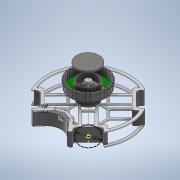
# Autodesk Inventor part: main_robot_backup
Saved by Autodesk Inventor 2020 (Build 240168000, 168)
## iProperties
Created: 2023-10-28
Part Number: main_robot_backup
Material: Типовые
Document SubType Name: Modeling
Designer: denis
Density: 1 g/cm^3
Appearance: По умолчанию
Mass: 193.225 g
Surface Area: 1128.99 cm^2
Volume: 193.225 cm^3
Author: denis
Autodesk Inventor part; units mm, degrees
(part 1 of 3)
sketch "bottom_frame" plane through (0, 0, 0) normal (0, 1, 0) x (-1, 0, 0)
  arc A0 (48.7014, 93.0224) -> (45.42, 94.668) centre (0, 0) ccw
  line L0 (0, 0) -> (74.2462, 74.2462) construction
  line L1 (85.2064, 46.3155) -> (87.5645, 48.6736)
  arc A1 (73.8927, 46.3155) -> (85.2064, 46.3155) centre (79.5495, 51.9723) ccw
  circle A2 centre (0, 0) radius 35 construction
  arc A3 (85.2064, -46.3155) -> (73.8927, -46.3155) centre (79.5495, -51.9723) ccw
  line L2 (85.2064, -46.3155) -> (87.5645, -48.6736)
  arc A4 (92.5543, -49.5852) -> (92.5543, 49.5852) centre (0, 0) ccw
  arc A5 (-46.3155, 73.8927) -> (-46.3155, 85.2064) centre (-51.9723, 79.5495) ccw
  line L3 (-48.6736, 87.5645) -> (-46.3155, 85.2064)
  arc A6 (-45.42, 94.668) -> (-48.7014, 93.0224) centre (0, 0) ccw
  arc A7 (46.3155, 85.2064) -> (46.3155, 73.8927) centre (51.9723, 79.5495) ccw
  line L4 (48.6736, 87.5645) -> (46.3155, 85.2064)
  arc A8 (44.0271, 95.3237) -> (43.577, 95.5303) centre (0, 0) ccw construction
  line L5 (46.3155, 73.8927) -> (73.8927, 46.3155)
  spline S0 degree 2 poles (87.5645, 48.6736) (91.1, 52.2091) (92.5543, 49.5852) knots 1 1 1 2 2 2
  line L6 (87.5645, 48.6736) -> (91.1, 52.2091) construction
  line L7 (91.1, 52.2091) -> (92.5543, 49.5852) construction
  line L8 (91.1, 52.2091) -> (87.5645, 48.6736) construction
  line L9 (87.5645, 48.6736) -> (91.1, 52.2091) construction
  line L10 (91.1, 52.2091) -> (92.5543, 49.5852) construction
  line L11 (91.1, 52.2091) -> (52.2091, 91.1) construction
  line L12 (52.2091, 91.1) -> (48.6736, 87.5645) construction
  line L13 (52.2091, 91.1) -> (48.6736, 87.5645) construction
  line L14 (48.6736, 87.5645) -> (52.2091, 91.1) construction
  spline S1 degree 2 poles (48.6736, 87.5645) (52.2091, 91.1) (48.7014, 93.0224) knots 1 1 1 2 2 2
  line L15 (52.2091, 91.1) -> (48.7014, 93.0224) construction
  line L16 (52.2091, 91.1) -> (48.7014, 93.0224) construction
  arc A9 (92.5543, 49.5852) -> (48.7014, 93.0224) centre (0, 0) ccw construction
  arc A10 (-85.2064, 46.3155) -> (-73.8927, 46.3155) centre (-79.5495, 51.9723) ccw
  line L17 (-85.2064, 46.3155) -> (-87.5645, 48.6736)
  spline S2 degree 2 poles (-48.6736, -87.5645) (-52.2091, -91.1) (-48.7014, -93.0224) knots 1 1 1 2 2 2
  line L18 (-48.6736, -87.5645) -> (-52.2091, -91.1) construction
  line L19 (-52.2091, -91.1) -> (-48.7014, -93.0224) construction
  line L20 (-48.6736, -87.5645) -> (-46.3155, -85.2064)
  line L21 (-46.3155, -73.8927) -> (-73.8927, -46.3155)
  arc A11 (-73.8927, -46.3155) -> (-85.2064, -46.3155) centre (-79.5495, -51.9723) ccw
  spline S3 degree 2 poles (-87.5645, -48.6736) (-91.1, -52.2091) (-92.5543, -49.5852) knots 1 1 1 2 2 2
  line L22 (-87.5645, -48.6736) -> (-91.1, -52.2091) construction
  line L23 (-91.1, -52.2091) -> (-92.5543, -49.5852) construction
  arc A12 (-92.5543, 49.5852) -> (-92.5543, -49.5852) centre (0, 0) ccw
  arc A13 (-92.5543, -49.5852) -> (-48.7014, -93.0224) centre (0, 0) ccw construction
  line L24 (-85.2064, -46.3155) -> (-87.5645, -48.6736)
  spline S4 degree 2 poles (-48.6736, 87.5645) (-52.2091, 91.1) (-48.7014, 93.0224) knots 1 1 1 2 2 2
  line L25 (-48.6736, 87.5645) -> (-52.2091, 91.1) construction
  line L26 (-52.2091, 91.1) -> (-48.7014, 93.0224) construction
  line L27 (-46.3155, 73.8927) -> (-73.8927, 46.3155)
  spline S5 degree 2 poles (-87.5645, 48.6736) (-91.1, 52.2091) (-92.5543, 49.5852) knots 1 1 1 2 2 2
  line L28 (-87.5645, 48.6736) -> (-91.1, 52.2091) construction
  line L29 (-91.1, 52.2091) -> (-92.5543, 49.5852) construction
  arc A14 (-48.7014, 93.0224) -> (-92.5543, 49.5852) centre (0, 0) ccw construction
  spline S6 degree 2 poles (48.6736, -87.5645) (52.2091, -91.1) (48.7014, -93.0224) knots 1 1 1 2 2 2
  line L30 (48.6736, -87.5645) -> (52.2091, -91.1) construction
  line L31 (52.2091, -91.1) -> (48.7014, -93.0224) construction
  line L32 (48.6736, -87.5645) -> (46.3155, -85.2064)
  arc A15 (46.3155, -73.8927) -> (46.3155, -85.2064) centre (51.9723, -79.5495) ccw
  line L33 (46.3155, -73.8927) -> (73.8927, -46.3155)
  spline S7 degree 2 poles (87.5645, -48.6736) (91.1, -52.2091) (92.5543, -49.5852) knots 1 1 1 2 2 2
  line L34 (87.5645, -48.6736) -> (91.1, -52.2091) construction
  line L35 (91.1, -52.2091) -> (92.5543, -49.5852) construction
  arc A16 (48.7014, -93.0224) -> (92.5543, -49.5852) centre (0, 0) ccw construction
  arc A17 (-46.3155, -85.2064) -> (-46.3155, -73.8927) centre (-51.9723, -79.5495) ccw
  arc A18 (-48.7014, -93.0224) -> (48.7014, -93.0224) centre (0, 0) ccw
  line L36 (43.0355, 94.1655) -> (18.3802, 65.3664)
  line L37 (17.477, 64.7643) -> (0.6161, 59.3045)
  line L38 (0, 0) -> (0, 95.3237) construction
  line L39 (-17.477, 64.7643) -> (-0.6161, 59.3045)
  line L40 (-43.0355, 94.1655) -> (-18.3802, 65.3664)
  arc A19 (45.42, 94.668) -> (43.0355, 94.1655) centre (44.5548, 92.8648) ccw
  arc A20 (17.477, 64.7643) -> (18.3802, 65.3664) centre (16.8609, 66.6671) ccw
  arc A21 (-0.6161, 59.3045) -> (0.6161, 59.3045) centre (0, 61.2072) ccw
  arc A22 (91.2033, 35.8602) -> (-91.2033, 35.8602) centre (0, 0) ccw construction
  line L41 (76.014, 34.2947) -> (37.1244, 73.1843)
  line L42 (87.156, 38.3657) -> (83.085, 34.2947)
  line L43 (22.4142, 59.3148) -> (25.4187, 62.8242) construction
  line L44 (21.5111, 58.7128) -> (14.5119, 56.4463) construction
  arc A23 (21.5111, 58.7128) -> (22.4142, 59.3148) centre (20.8949, 60.6155) ccw
  line L45 (-14.5119, 56.4463) -> (-0.6161, 51.9466)
  line L46 (-25.4187, 62.8242) -> (-34.1909, 73.0707)
  arc A24 (-0.6161, 51.9466) -> (0.6161, 51.9466) centre (0, 53.8493) ccw
  arc A25 (37.1244, 73.1843) -> (34.1909, 73.0707) centre (35.7102, 71.7701) ccw
  arc A26 (-22.4142, 59.3148) -> (-21.5111, 58.7128) centre (-20.8949, 60.6155) ccw
  line L47 (90.4123, 37.7305) -> (91.2033, 35.8602)
  arc A27 (90.4123, 37.7305) -> (87.156, 38.3657) centre (88.5702, 36.9514) ccw
  arc A28 (85.9577, -47.0668) -> (91.2033, -35.8602) centre (0, 0) ccw construction
  arc A29 (-87.156, 38.3657) -> (-90.4123, 37.7305) centre (-88.5702, 36.9514) ccw
  line L48 (-90.4123, 37.7305) -> (-91.2033, 35.8602)
  line L49 (-87.156, 38.3657) -> (-83.085, 34.2947)
  line L50 (-76.014, 34.2947) -> (-37.1244, 73.1843)
  arc A30 (-34.1909, 73.0707) -> (-37.1244, 73.1843) centre (-35.7102, 71.7701) ccw
  arc A31 (-91.2033, 35.8602) -> (-91.2033, -35.8602) centre (0, 0) ccw
  line L51 (76.014, -34.2947) -> (34.2947, -76.014)
  line L52 (46.3155, -73.8927) -> (73.8927, -46.3155) construction
  line L53 (87.156, -38.3657) -> (83.085, -34.2947)
  line L54 (38.3657, -87.156) -> (34.2947, -83.085)
  line L55 (48.6736, -87.5645) -> (46.3155, -85.2064) construction
  line L56 (90.4123, -37.7305) -> (91.2033, -35.8602)
  arc A32 (87.156, -38.3657) -> (90.4123, -37.7305) centre (88.5702, -36.9514) ccw
  arc A33 (83.085, -34.2947) -> (76.014, -34.2947) centre (79.5495, -37.8302) ccw
  arc A34 (34.2947, -76.014) -> (34.2947, -83.085) centre (37.8302, -79.5495) ccw
  line L57 (37.7305, -90.4123) -> (35.8602, -91.2033)
  arc A35 (37.7305, -90.4123) -> (38.3657, -87.156) centre (36.9514, -88.5702) ccw
  line L58 (-34.2947, -76.014) -> (-76.014, -34.2947)
  line L59 (-73.8927, -46.3155) -> (-46.3155, -73.8927) construction
  line L60 (-34.2947, -83.085) -> (-38.3657, -87.156)
  line L61 (-46.3155, -85.2064) -> (-48.6736, -87.5645) construction
  line L62 (-83.085, -34.2947) -> (-87.156, -38.3657)
  arc A36 (-34.2947, -83.085) -> (-34.2947, -76.014) centre (-37.8302, -79.5495) ccw
  arc A37 (-76.014, -34.2947) -> (-83.085, -34.2947) centre (-79.5495, -37.8302) ccw
  line L63 (-37.7305, -90.4123) -> (-35.8602, -91.2033)
  arc A38 (-38.3657, -87.156) -> (-37.7305, -90.4123) centre (-36.9514, -88.5702) ccw
  line L64 (-90.4123, -37.7305) -> (-91.2033, -35.8602)
  arc A39 (-90.4123, -37.7305) -> (-87.156, -38.3657) centre (-88.5702, -36.9514) ccw
  arc A40 (-91.2033, -35.8602) -> (-35.8602, -91.2033) centre (0, 0) ccw construction
  arc A41 (-35.8602, -91.2033) -> (35.8602, -91.2033) centre (0, 0) ccw
  arc A42 (35.8602, -91.2033) -> (85.9577, -47.0668) centre (0, 0) ccw construction
  arc A43 (91.2033, -35.8602) -> (91.2033, 35.8602) centre (0, 0) ccw
  line L65 (-34.1909, 73.0707) -> (-27.0558, 64.7365) construction
  arc A44 (-43.0355, 94.1655) -> (-45.42, 94.668) centre (-44.5548, 92.8648) ccw
  arc A45 (-18.3802, 65.3664) -> (-17.477, 64.7643) centre (-16.8609, 66.6671) ccw
  line L66 (-76.014, -34.2947) -> (-34.2947, -76.014) construction
  line L67 (0, 0) -> (60.1041, -60.1041) construction
  line L68 (73.8927, -46.3155) -> (46.3155, -73.8927) construction
  line L69 (37.4767, -12.0208) -> (67.8823, -42.4264)
  line L70 (42.4264, -67.8823) -> (12.0208, -37.4767)
  line L71 (33.9411, -19.799) -> (19.799, -33.9411)
  line L72 (34.6482, -12.0208) -> (12.0208, -34.6482)
  line L73 (36.7696, -19.799) -> (63.6396, -46.669)
  line L74 (19.799, -36.7696) -> (46.669, -63.6396)
  arc A46 (36.7696, -19.799) -> (33.9411, -19.799) centre (35.3553, -21.2132) ccw
  arc A47 (19.799, -33.9411) -> (19.799, -36.7696) centre (21.2132, -35.3553) ccw
  arc A48 (12.0208, -34.6482) -> (12.0208, -37.4767) centre (13.435, -36.0624) ccw construction
  arc A49 (37.4767, -12.0208) -> (34.6482, -12.0208) centre (36.0624, -13.435) ccw construction
  line L75 (98, 0) -> (-98, 0) construction
  line L76 (37.4767, 12.0208) -> (67.8823, 42.4264)
  line L77 (36.7696, 19.799) -> (63.6396, 46.669)
  line L78 (34.6482, 12.0208) -> (13.1066, 33.5624)
  arc A50 (33.9411, 19.799) -> (36.7696, 19.799) centre (35.3553, 21.2132) ccw
  arc A51 (34.6482, 12.0208) -> (37.4767, 12.0208) centre (36.0624, 13.435) ccw construction
  line L79 (33.9411, 19.799) -> (19.799, 33.9411)
  arc A52 (19.799, 36.7696) -> (19.799, 33.9411) centre (21.2132, 35.3553) ccw
  arc A53 (12.0208, 37.4767) -> (12.0208, 34.6482) centre (13.435, 36.0624) ccw construction
  line L80 (42.4264, 67.8823) -> (12.0208, 37.4767)
  line L81 (19.799, 36.7696) -> (46.669, 63.6396)
  line L82 (-19.799, -36.7696) -> (-46.669, -63.6396)
  line L83 (-36.7696, -19.799) -> (-63.6396, -46.669)
  line L84 (-37.4767, -12.0208) -> (-67.8823, -42.4264)
  arc A54 (-19.799, -36.7696) -> (-19.799, -33.9411) centre (-21.2132, -35.3553) ccw
  arc A55 (-33.9411, -19.799) -> (-36.7696, -19.799) centre (-35.3553, -21.2132) ccw
  arc A56 (-12.0208, -37.4767) -> (-12.0208, -34.6482) centre (-13.435, -36.0624) ccw construction
  arc A57 (-34.6482, -12.0208) -> (-37.4767, -12.0208) centre (-36.0624, -13.435) ccw construction
  line L85 (-33.9411, -19.799) -> (-19.799, -33.9411)
  line L86 (-34.6482, -12.0208) -> (-12.0208, -34.6482)
  line L87 (-42.4264, -67.8823) -> (-12.0208, -37.4767)
  arc A58 (-12.0208, 34.6482) -> (-12.0208, 37.4767) centre (-13.435, 36.0624) ccw construction
  line L88 (-19.799, 36.7696) -> (-46.669, 63.6396)
  line L89 (-42.4264, 67.8823) -> (-12.0208, 37.4767)
  arc A59 (-19.799, 33.9411) -> (-19.799, 36.7696) centre (-21.2132, 35.3553) ccw
  line L90 (-33.9411, 19.799) -> (-19.799, 33.9411)
  line L91 (-34.6482, 12.0208) -> (-12.0208, 34.6482)
  arc A60 (-36.7696, 19.799) -> (-33.9411, 19.799) centre (-35.3553, 21.2132) ccw
  arc A61 (-37.4767, 12.0208) -> (-34.6482, 12.0208) centre (-36.0624, 13.435) ccw construction
  line L92 (-37.4767, 12.0208) -> (-67.8823, 42.4264)
  line L93 (-36.7696, 19.799) -> (-63.6396, 46.669)
  line L94 (37.4767, 12.0208) -> (-12.0208, -37.4767) construction
  line L95 (12.0208, 37.4767) -> (-37.4767, -12.0208) construction
  line L96 (12.0208, -37.4767) -> (-37.4767, 12.0208) construction
  line L97 (37.4767, -12.0208) -> (-12.0208, 37.4767) construction
  line L98 (14.1421, -32.5269) -> (-32.5269, 14.1421) construction
  line L99 (32.5269, -14.1421) -> (-14.1421, 32.5269) construction
  line L100 (14.1421, 32.5269) -> (-32.5269, -14.1421) construction
  line L101 (32.5269, 14.1421) -> (-14.1421, -32.5269) construction
  line L102 (38.5624, -11.7401) -> (33.5624, -11.7401) construction
  line L103 (33.5624, -13.1066) -> (33.5624, 13.1066)
  line L104 (33.5624, 10.7237) -> (38.5624, 10.7237) construction
  line L105 (38.5624, 13.1066) -> (38.5624, -13.1066)
  line L106 (36.0624, -11.7401) -> (36.0624, 10.7237) construction
  line L107 (36.0624, -13.435) -> (36.0624, 13.435) construction
  line L108 (-38.5624, 13.1066) -> (-38.5624, -13.1066)
  line L109 (-33.5624, -13.1066) -> (-33.5624, 13.1066)
  line L110 (-13.1066, -38.5624) -> (13.1066, -38.5624)
  line L111 (13.1066, -33.5624) -> (-13.1066, -33.5624)
  line L112 (13.1066, 38.5624) -> (-13.1066, 38.5624)
  line L113 (-13.1066, 33.5624) -> (13.1066, 33.5624)
  line L114 (0, 51.8493) -> (0, 56.3493) construction
  line L115 (-2.0518, 60.1742) -> (-0.6251, 60.6437)
  line L116 (0.6251, 60.6437) -> (2.0518, 60.1742)
  line L117 (2.672, 59.9702) -> (4.5, 60.5621) construction
  line L118 (-2.672, 59.9702) -> (-4.5, 60.5621) construction
  arc A62 (0.6251, 60.6437) -> (-0.6251, 60.6437) centre (0, 58.7439) ccw
  arc A63 (2.0518, 60.1742) -> (3.2931, 60.1713) centre (2.6769, 62.074) ccw
  arc A64 (-3.2931, 60.1713) -> (-2.0518, 60.1742) centre (-2.6769, 62.074) ccw
  arc A65 (2.672, 59.9702) -> (2.5156, 60.0805) centre (0, 56.3493) ccw construction
  arc A66 (-2.5156, 60.0805) -> (-2.672, 59.9702) centre (0, 56.3493) ccw construction
  arc A67 (0, 51.8493) -> (0.3604, 51.8638) centre (0, 56.3493) ccw construction
  arc A68 (1.5976, 52.1425) -> (2.3373, 52.504) centre (0, 56.3493) ccw construction
  arc A69 (76.014, 34.2947) -> (83.085, 34.2947) centre (79.5495, 37.8302) ccw
  arc A70 (-83.085, 34.2947) -> (-76.014, 34.2947) centre (-79.5495, 37.8302) ccw
  line L119 (0, 105) -> (0, 104.941) construction
  line L120 (0, 104.941) -> (-23.6028, 54.3247) construction
  line L121 (0, 104.941) -> (-20.5578, 60.8546) construction
  circle A71 centre (-20.5578, 60.8546) radius 1.55
  line L122 (-20.5578, 60.8546) -> (-22.0043, 58.9513) construction
  line L123 (-20.5578, 60.8546) -> (-24.1768, 56.0927) construction
  line L124 (-15.1585, 56.5907) -> (-21.0049, 57.3328)
  line L125 (-24.842, 61.8893) -> (-23.8313, 59.4808)
  arc A72 (-24.842, 61.8893) -> (-25.4187, 62.8242) centre (-28.1154, 60.5155) ccw
  arc A73 (-14.5119, 56.4463) -> (-15.1585, 56.5907) centre (-15.6055, 53.069) ccw
  arc A74 (-23.8313, 59.4808) -> (-21.0049, 57.3328) centre (-20.5578, 60.8546) ccw
  line L126 (15.1585, 56.5907) -> (21.0049, 57.3328)
  line L127 (24.842, 61.8893) -> (23.8313, 59.4808)
  arc A75 (25.4187, 62.8242) -> (24.842, 61.8893) centre (28.1154, 60.5155) ccw
  arc A76 (15.1585, 56.5907) -> (14.5119, 56.4463) centre (15.6055, 53.069) ccw
  arc A77 (21.0049, 57.3328) -> (23.8313, 59.4808) centre (20.5578, 60.8546) ccw
  line L128 (25.4187, 62.8242) -> (34.1909, 73.0707)
  line L129 (14.5119, 56.4463) -> (0.6161, 51.9466)
  circle A78 centre (20.5578, 60.8546) radius 1.55
  line L130 (13.1066, 33.5624) -> (12.0208, 34.6482)
  point P0 (40.6586, 79.5495)
  point P1 (60.1041, 60.1041)
  point P2 (79.5495, 40.6586)
  point P3 (-43.577, 95.5303)
  point P4 (18.0135, 64.938)
  point P5 (0, 59.1049)
  point P6 (-18.0135, 64.938)
  point P7 (-44.0271, 95.3237)
  point P8 (79.5495, 30.7591)
  point P9 (55.1543, 55.1543)
  point P10 (89.2556, 40.4652)
  point P11 (27.0558, 64.7365)
  point P12 (0, 51.7471)
  point P13 (89.2556, 40.4652)
  point P14 (79.5495, 30.7591)
  point P15 (35.5963, 74.7124)
  point P16 (80.9637, 32.1734)
  point P17 (78.1353, 32.1734)
  point P18 (0, 66.2072)
  point P19 (-80.9637, 32.1734)
  point P20 (-78.1353, 32.1734)
  point P21 (89.2556, -40.4652)
  point P22 (40.4652, -89.2556)
  point P23 (-40.4652, -89.2556)
  point P24 (-89.2556, -40.4652)
  point P25 (-60.1041, -60.1041)
  point P26 (-55.1543, 55.1543)
  point P27 (-60.1041, 60.1041)
  point P28 (0, 59.2072)
  point P29 (-39.283, 89.7822)
  point P30 (-38.5624, -13.1066)
  point P31 (-33.5624, 13.1066)
  point P32 (-23.0382, 57.5909)
  point P33 (-22.7059, 58.0282)
  point P34 (-21.4957, 59.6205)
  dimension "d208" = 3.1
  dimension "d29" = 16.3348
  dimension "d30" = 27.5
  dimension "d31" = 8
  dimension "d32" = 5
  dimension "d33" = 5
  dimension "d34" = 3
  dimension "d35" = 4
  dimension "d36" = 70
  dimension "d37" = 85
  dimension "d38" = 105
  dimension "d39" = 40
  dimension "d40" = 18.9344
  dimension "d41" = 5.21
  dimension "d42" = 2
  dimension "d43" = 7
  dimension "d44" = 7
  dimension "d45" = 7
  dimension "d46" = 7
  dimension "d47" = 7
  dimension "d48" = 2
  dimension "d49" = 2
  dimension "d50" = 2
  dimension "d51" = 5
  dimension "d52" = 2
  dimension "d53" = 7
  dimension "d54" = 7
  dimension "d55" = 7
  dimension "d56" = 5
  dimension "d57" = 2
  dimension "d58" = 5
  dimension "d59" = 5
  dimension "d60" = 2
  dimension "d61" = 7
  dimension "d62" = 7
  dimension "d63" = 7
  dimension "d64" = 5
  dimension "d65" = 5
  dimension "d66" = 2
  dimension "d67" = 5
  dimension "d68" = 2
  dimension "d69" = 2
  dimension "d70" = 40
  dimension "d71" = 5
  dimension "d72" = 6
  dimension "d73" = 6
  dimension "d74" = 12
  dimension "d75" = 12
  dimension "d76" = 2
  dimension "d77" = 5
  dimension "d78" = 5
  dimension "d79" = 5
  dimension "d80" = 5
  dimension "d81" = 7
  dimension "d82" = 5
  dimension "d160" = 4.5
  dimension "d163" = 2
  dimension "d200" = 5
  dimension "d201" = 5
  dimension "d205" = 0.059
  dimension "d206" = 25
  dimension "d207" = 48.644
  dimension "d216" = 40.567
  dimension "d217" = 1.7087
  dimension "d219" = 120
  constraints: 230 end point, 180 point on circle, 91 symmetric about line, 82 point on line, 77 centre point, 66 tangent, 27 parallel, 18 coincident, 12 equal radius, 5 perpendicular, 4 collinear, 4 midpoint, 2 vertical, 1 horizontal, 70 other
  measures "d29" distance of L8.start point (79.55, 40.659)
  measures "d30" distance of point (40.659, 79.55) point (60.104, 60.104)
  measures "d31" radius of A7
  measures "d32" distance of L12.start L4.start
  measures "d33" distance of L1.end L8.start
  measures "d34" distance of L8.start L7.end
  measures "d35" distance of L12.start L15.end
  measures "d36" diameter of A2
  measures "d37" distance of point (60.104, 60.104) L0.start
  measures "d38" radius of A4
  measures "d39" distance of A8.start point (18.013, 64.938)
  measures "d40" distance of point (18.013, 64.938) point (0, 59.105)
  measures "d41" distance of A8.start L15.end
  measures "d42" radius of A19
  measures "d43" radial gap between concentric circles of A4 A22
  measures "d44" distance between parallel lines of L5 L41
  measures "d45" distance between parallel lines of L1 L42
  measures "d46" distance between parallel lines of L43 L36
  measures "d47" distance between parallel lines of L37 L44
  measures "d48" radius of A23
  measures "d49" radius of A24
  measures "d50" radius of A25
  measures "d51" distance of point (89.256, 40.465) L47.end
  measures "d52" radius of A27
  measures "d53" distance between parallel lines of L53 L2
  measures "d54" distance between parallel lines of L32 L54
  measures "d55" distance between parallel lines of L51 L33
  measures "d56" distance of point (89.256, -40.465) L56.end
  measures "d57" radius of A32
  measures "d58" radius of A33
  measures "d59" distance of point (40.465, -89.256) L57.end
  measures "d60" radius of A35
  measures "d61" distance between parallel lines of L21 L58
  measures "d62" distance between parallel lines of L20 L60
  measures "d63" distance between parallel lines of L24 L62
  measures "d64" radius of A36
  measures "d65" distance of point (-40.465, -89.256) L63.end
  measures "d66" radius of A38
  measures "d67" distance of point (-89.256, -40.465) L64.end
  measures "d68" radius of A39
  measures "d69" radius of A44
  measures "d70" distance between parallel lines of L71 L51
  measures "d71" distance between parallel lines of L71 L72
  measures "d72" distance between parallel lines of L69 L73
  measures "d73" distance between parallel lines of L70 L74
  measures "d74" distance between parallel lines of L67 L74
  measures "d75" distance between parallel lines of L73 L67
  measures "d76" radius of A46
  measures "d77" distance between parallel lines of L96 L98
  measures "d78" distance between parallel lines of L97 L99
  measures "d79" distance between parallel lines of L95 L100
  measures "d80" distance between parallel lines of L94 L101
  measures "d81" distance of point (0, 66.207) point (0, 59.207)
  measures "d82" distance between parallel lines of L103 L105
  measures "d160" distance of L114.start L114.end
  measures "d163" radius of A62
  measures "d200" radius of A69
  measures "d201" radius of A70
  measures "d205" distance of L119.start L119.end
  measures "d206" angle of L38 L120
  measures "d207" distance of L119.end L121.end
  measures "d216" angle of L36 L38
  measures "d217" distance of L122.end point (-23.038, 57.591)
  measures "d219" angle of L125 L124
sketch "motowheels" plane through (0, 0, 0) normal (0, 1, 0) x (-1, 0, 0)
  line L0 (0, 0) -> (-79.4987, -79.4987) construction
  line L1 (-21.7082, -36.1332) -> (-50.7703, -65.1952) construction
  line L2 (-50.7703, -65.1952) -> (-65.1952, -50.7703) construction
  line L3 (-65.1952, -50.7703) -> (-36.1332, -21.7082) construction
  line L4 (-36.1332, -21.7082) -> (-21.7082, -36.1332) construction
  line L5 (-28.9207, -28.9207) -> (-57.9828, -57.9828) construction
  line L6 (-69.8885, -50.3196) -> (-42.3114, -77.8968) construction
  line L7 (-57.6292, -62.579) -> (-55.5079, -60.4576) construction
  line L8 (-55.5079, -60.4576) -> (-60.4576, -55.5079) construction
  line L9 (-60.4576, -55.5079) -> (-62.579, -57.6292) construction
  line L10 (-62.579, -57.6292) -> (-57.6292, -62.579) construction
  line L11 (-57.9828, -57.9828) -> (-60.1041, -60.1041) construction
  line L12 (-58.8666, -61.3415) -> (-69.4732, -71.9481) construction
  line L13 (-69.4732, -71.9481) -> (-71.9481, -69.4732) construction
  line L14 (-71.9481, -69.4732) -> (-61.3415, -58.8666) construction
  line L15 (-61.3415, -58.8666) -> (-58.8666, -61.3415) construction
  line L16 (-60.1041, -60.1041) -> (-70.7107, -70.7107) construction
  line L17 (-44.5477, -79.9031) -> (-49.4975, -84.8528) construction
  line L18 (-49.4975, -84.8528) -> (-84.8528, -49.4975) construction
  line L19 (-84.8528, -49.4975) -> (-79.9031, -44.5477) construction
  line L20 (-79.9031, -44.5477) -> (-44.5477, -79.9031) construction
  line L21 (-67.1751, -67.1751) -> (-62.2254, -62.2254) construction
  arc A0 (-51.9723, -82.3779) -> (-47.0226, -77.4282) centre (-49.4975, -79.9031) ccw
  arc A1 (-77.4282, -47.0226) -> (-82.3779, -51.9723) centre (-79.9031, -49.4975) ccw
  line L22 (0, 0) -> (74.2462, 74.2462) construction
  line L23 (-46.3155, -73.8927) -> (-73.8927, -46.3155) projected
  line L24 (0, 0) -> (0, 95.3237) construction
  arc A2 (47.0226, -77.4282) -> (51.9723, -82.3779) centre (49.4975, -79.9031) ccw
  line L25 (44.5477, -79.9031) -> (49.4975, -84.8528) construction
  line L26 (0, 0) -> (79.4987, -79.4987) construction
  line L27 (21.7082, -36.1332) -> (50.7703, -65.1952) construction
  line L28 (50.7703, -65.1952) -> (65.1952, -50.7703) construction
  line L29 (65.1952, -50.7703) -> (36.1332, -21.7082) construction
  line L30 (36.1332, -21.7082) -> (21.7082, -36.1332) construction
  line L31 (28.9207, -28.9207) -> (57.9828, -57.9828) construction
  line L32 (69.8885, -50.3196) -> (42.3114, -77.8968) construction
  line L33 (57.6292, -62.579) -> (55.5079, -60.4576) construction
  line L34 (61.3415, -58.8666) -> (58.8666, -61.3415) construction
  line L35 (57.9828, -57.9828) -> (60.1041, -60.1041) construction
  line L36 (69.4732, -71.9481) -> (71.9481, -69.4732) construction
  line L37 (67.1751, -67.1751) -> (62.2254, -62.2254) construction
  line L38 (62.579, -57.6292) -> (57.6292, -62.579) construction
  line L39 (55.5079, -60.4576) -> (60.4576, -55.5079) construction
  line L40 (58.8666, -61.3415) -> (69.4732, -71.9481) construction
  line L41 (60.1041, -60.1041) -> (70.7107, -70.7107) construction
  line L42 (49.4975, -84.8528) -> (84.8528, -49.4975) construction
  line L43 (79.9031, -44.5477) -> (44.5477, -79.9031) construction
  line L44 (71.9481, -69.4732) -> (61.3415, -58.8666) construction
  line L45 (60.4576, -55.5079) -> (62.579, -57.6292) construction
  arc A3 (82.3779, -51.9723) -> (77.4282, -47.0226) centre (79.9031, -49.4975) ccw
  line L46 (84.8528, -49.4975) -> (79.9031, -44.5477) construction
  line L47 (46.3155, -73.8927) -> (73.8927, -46.3155)
  line L48 (98, 0) -> (-98, 0) construction
  arc A4 (-47.0226, 77.4282) -> (-51.9723, 82.3779) centre (-49.4975, 79.9031) ccw
  line L49 (-44.5477, 79.9031) -> (-49.4975, 84.8528) construction
  line L50 (0, 0) -> (-79.4987, 79.4987) construction
  line L51 (-21.7082, 36.1332) -> (-50.7703, 65.1952) construction
  line L52 (-50.7703, 65.1952) -> (-65.1952, 50.7703) construction
  line L53 (-65.1952, 50.7703) -> (-36.1332, 21.7082) construction
  line L54 (-36.1332, 21.7082) -> (-21.7082, 36.1332) construction
  line L55 (-28.9207, 28.9207) -> (-57.9828, 57.9828) construction
  line L56 (-69.8885, 50.3196) -> (-42.3114, 77.8968) construction
  line L57 (-57.6292, 62.579) -> (-55.5079, 60.4576) construction
  line L58 (-61.3415, 58.8666) -> (-58.8666, 61.3415) construction
  line L59 (-57.9828, 57.9828) -> (-60.1041, 60.1041) construction
  line L60 (-69.4732, 71.9481) -> (-71.9481, 69.4732) construction
  line L61 (-67.1751, 67.1751) -> (-62.2254, 62.2254) construction
  line L62 (-62.579, 57.6292) -> (-57.6292, 62.579) construction
  line L63 (-55.5079, 60.4576) -> (-60.4576, 55.5079) construction
  line L64 (-58.8666, 61.3415) -> (-69.4732, 71.9481) construction
  line L65 (-60.1041, 60.1041) -> (-70.7107, 70.7107) construction
  line L66 (-49.4975, 84.8528) -> (-84.8528, 49.4975) construction
  line L67 (-79.9031, 44.5477) -> (-44.5477, 79.9031) construction
  line L68 (-71.9481, 69.4732) -> (-61.3415, 58.8666) construction
  line L69 (-60.4576, 55.5079) -> (-62.579, 57.6292) construction
  arc A5 (-82.3779, 51.9723) -> (-77.4282, 47.0226) centre (-79.9031, 49.4975) ccw
  line L70 (-84.8528, 49.4975) -> (-79.9031, 44.5477) construction
  line L71 (-46.3155, 73.8927) -> (-73.8927, 46.3155)
  arc A6 (77.4282, 47.0226) -> (82.3779, 51.9723) centre (79.9031, 49.4975) ccw
  line L72 (84.8528, 49.4975) -> (79.9031, 44.5477) construction
  line L73 (58.8666, 61.3415) -> (69.4732, 71.9481) construction
  line L74 (67.1751, 67.1751) -> (62.2254, 62.2254) construction
  line L75 (0, 0) -> (79.4987, 79.4987) construction
  line L76 (21.7082, 36.1332) -> (50.7703, 65.1952) construction
  line L77 (65.1952, 50.7703) -> (36.1332, 21.7082) construction
  line L78 (28.9207, 28.9207) -> (57.9828, 57.9828) construction
  line L79 (60.4576, 55.5079) -> (62.579, 57.6292) construction
  line L80 (61.3415, 58.8666) -> (58.8666, 61.3415) construction
  line L81 (57.9828, 57.9828) -> (60.1041, 60.1041) construction
  line L82 (69.4732, 71.9481) -> (71.9481, 69.4732) construction
  line L83 (62.579, 57.6292) -> (57.6292, 62.579) construction
  line L84 (55.5079, 60.4576) -> (60.4576, 55.5079) construction
  line L85 (71.9481, 69.4732) -> (61.3415, 58.8666) construction
  line L86 (57.6292, 62.579) -> (55.5079, 60.4576) construction
  line L87 (60.1041, 60.1041) -> (70.7107, 70.7107) construction
  line L88 (50.7703, 65.1952) -> (65.1952, 50.7703) construction
  line L89 (49.4975, 84.8528) -> (84.8528, 49.4975) construction
  line L90 (79.9031, 44.5477) -> (44.5477, 79.9031) construction
  line L91 (46.3155, 73.8927) -> (73.8927, 46.3155)
  line L92 (69.8885, 50.3196) -> (42.3114, 77.8968) construction
  arc A7 (51.9723, 82.3779) -> (47.0226, 77.4282) centre (49.4975, 79.9031) ccw
  line L93 (44.5477, 79.9031) -> (49.4975, 84.8528) construction
  line L94 (36.1332, 21.7082) -> (21.7082, 36.1332) construction
  point P0 (-56.0999, -64.1082)
  point P1 (56.0999, -64.1082)
  point P2 (-56.0999, 64.1082)
  point P3 (56.0999, 64.1082)
  dimension "d224" = 20.4
  dimension "d225" = 3
  dimension "d226" = 3
  dimension "d227" = 7
  dimension "d228" = 15
  dimension "d229" = 3.5
  dimension "d230" = 7
  dimension "d231" = 50
  dimension "d232" = 3
  dimension "d233" = 41.1
  constraints: 182 end point, 111 symmetric about line, 16 point on circle, 9 midpoint, 8 centre point, 8 collinear, 8 parallel, 8 point on line, 4 perpendicular, 3 tangent, 7 other
  measures "d224" distance of L1.end L2.end
  measures "d225" distance from line of L2 point (-56.1, -64.108)
  measures "d226" distance of L7.start L7.end
  measures "d227" distance of L8.end L7.end
  measures "d228" distance of L15.end L13.start
  measures "d229" distance of L13.start L13.end
  measures "d230" distance of L17.start L17.end
  measures "d231" distance of L17.end L18.end
  measures "d232" distance between parallel lines of L10 L20
  measures "d233" distance of L2.end L3.end
sketch "Эскиз1" plane through (0, 0, 0) normal (0, 1, 0) x (-1, 0, 0)
  arc A0 (43.577, 95.5303) -> (-43.577, 95.5303) centre (0, 0) ccw construction
  line L0 (0, 0) -> (0, 209.8821) construction
  arc A1 (23.7825, 76.5969) -> (0, 67.941) centre (0, 104.941) ccw construction
  line L1 (0, 56.6418) -> (23.7825, 76.5969) construction
  line L2 (0, 56.6418) -> (-35.5516, 86.4744) construction
  line L3 (44.0271, 95.3237) -> (44.0271, 127.8162) construction
  ellipse E0 centre (0, 102.7511) end of major axis (44.0271, 102.7511) minor radius 27.5932 (42.0492, 94.5734) -> (35.2734, 86.2384) ccw construction
  line L4 (42.6652, 95.941) -> (-42.6652, 95.941) construction
  line L5 (0, 0) -> (74.2462, 74.2462) construction
  line L6 (44.1942, 76.014) -> (76.014, 44.1942) construction
  line L7 (83.085, 44.1942) -> (87.5645, 48.6736) construction
  line L8 (91.1, 52.2091) -> (52.2091, 91.1) construction
  line L9 (52.2091, 91.1) -> (48.6736, 87.5645) construction
  arc A2 (44.1942, 83.085) -> (44.1942, 76.014) centre (47.7297, 79.5495) ccw construction
  arc A3 (76.014, 44.1942) -> (83.085, 44.1942) centre (79.5495, 47.7297) ccw construction
  line L10 (52.2091, 91.1) -> (48.6736, 87.5645) construction
  line L11 (42.6652, 95.941) -> (43.577, 95.5303) construction
  line L12 (42.6652, 95.941) -> (42.0492, 94.5734) construction
  line L13 (42.0492, 94.5734) -> (42.6652, 95.941) construction
  line L14 (42.6652, 95.941) -> (43.577, 95.5303) construction
  spline S0 degree 2 poles (42.0492, 94.5734) (42.6652, 95.941) (43.577, 95.5303) knots 1 1 1 2 2 2
  line L15 (-42.6652, 95.941) -> (-42.0492, 94.5734) construction
  line L16 (-42.6652, 95.941) -> (-43.577, 95.5303) construction
  line L17 (-42.0492, 94.5734) -> (-42.6652, 95.941) construction
  line L18 (-42.6652, 95.941) -> (-43.577, 95.5303) construction
  spline S1 degree 2 poles (-42.0492, 94.5734) (-42.6652, 95.941) (-43.577, 95.5303) knots 1 1 1 2 2 2 construction
  line L19 (52.2091, 91.1) -> (48.7014, 93.0224) construction
  line L20 (48.6736, 87.5645) -> (52.2091, 91.1) construction
  line L21 (52.2091, 91.1) -> (48.7014, 93.0224) construction
  spline S2 degree 2 poles (48.6736, 87.5645) (52.2091, 91.1) (48.7014, 93.0224) knots 1 1 1 2 2 2
  spline S3 degree 2 poles (-48.6736, 87.5645) (-52.2091, 91.1) (-48.7014, 93.0224) knots 1 1 1 2 2 2
  arc A4 (-44.1942, 76.014) -> (-44.1942, 83.085) centre (-47.7297, 79.5495) ccw
  line L22 (-44.1942, 76.014) -> (-76.014, 44.1942)
  arc A5 (-83.085, 44.1942) -> (-76.014, 44.1942) centre (-79.5495, 47.7297) ccw
  line L23 (-83.085, 44.1942) -> (-87.3563, 48.4654)
  line L24 (-48.6736, 87.5645) -> (-52.2091, 91.1) construction
  line L25 (-52.2091, 91.1) -> (-48.7014, 93.0224) construction
  spline S4 degree 2 poles (48.6736, -87.5645) (52.2091, -91.1) (48.7014, -93.0224) knots 1 1 1 2 2 2 construction
  line L26 (48.6736, -87.5645) -> (52.2091, -91.1) construction
  line L27 (52.2091, -91.1) -> (48.7014, -93.0224) construction
  line L28 (48.6736, -87.5645) -> (46.3155, -85.2064) construction
  arc A6 (46.3155, -73.8927) -> (46.3155, -85.2064) centre (51.9723, -79.5495) ccw construction
  line L29 (46.3155, -73.8927) -> (73.8927, -46.3155) construction
  arc A7 (85.2064, -46.3155) -> (73.8927, -46.3155) centre (79.5495, -51.9723) ccw construction
  line L30 (85.2064, -46.3155) -> (87.5645, -48.6736) construction
  spline S5 degree 2 poles (87.5645, -48.6736) (91.1, -52.2091) (92.5543, -49.5852) knots 1 1 1 2 2 2 construction
  line L31 (87.5645, -48.6736) -> (91.1, -52.2091) construction
  line L32 (91.1, -52.2091) -> (92.5543, -49.5852) construction
  spline S6 degree 2 poles (-48.6736, -87.5645) (-52.2091, -91.1) (-48.7014, -93.0224) knots 1 1 1 2 2 2 construction
  line L33 (-48.6736, -87.5645) -> (-52.2091, -91.1) construction
  line L34 (-52.2091, -91.1) -> (-48.7014, -93.0224) construction
  line L35 (-48.6736, -87.5645) -> (-46.3155, -85.2064) construction
  arc A8 (-46.3155, -85.2064) -> (-46.3155, -73.8927) centre (-51.9723, -79.5495) ccw construction
  line L36 (-46.3155, -73.8927) -> (-73.8927, -46.3155) construction
  arc A9 (-73.8927, -46.3155) -> (-85.2064, -46.3155) centre (-79.5495, -51.9723) ccw construction
  spline S7 degree 2 poles (-87.5645, -48.6736) (-91.1, -52.2091) (-92.5543, -49.5852) knots 1 1 1 2 2 2 construction
  line L37 (-87.5645, -48.6736) -> (-91.1, -52.2091) construction
  line L38 (-91.1, -52.2091) -> (-92.5543, -49.5852) construction
  line L39 (-85.2064, -46.3155) -> (-87.5645, -48.6736) construction
  ellipse E1 centre (0, 102.7511) end of major axis (44.5159, 105.2445) minor radius 28.887 (35.2734, 86.2384) -> (42.0492, 94.5734) ccw
  arc A10 (0, 67.941) -> (23.7825, 76.5969) centre (0, 104.941) ccw
  line L40 (23.7825, 76.5969) -> (35.2734, 86.2384)
  line L41 (-23.7825, 76.5969) -> (-35.2734, 86.2384)
  arc A11 (-23.7825, 76.5969) -> (0, 67.941) centre (0, 104.941) ccw
  ellipse E2 centre (0, 102.7511) end of major axis (-44.5159, 105.2445) minor radius 28.887 (-42.0492, 94.5734) -> (-35.2734, 86.2384) ccw
  spline S8 degree 2 poles (-42.0492, 94.5734) (-42.6652, 95.941) (-43.577, 95.5303) knots 1 1 1 2 2 2
  line L42 (-42.0492, 94.5734) -> (-42.6652, 95.941) construction
  line L43 (-42.6652, 95.941) -> (-43.577, 95.5303) construction
  arc A12 (44.0271, 95.3237) -> (43.577, 95.5303) centre (0, 0) ccw construction
  arc A13 (48.7014, 93.0224) -> (44.0271, 95.3237) centre (0, 0) ccw
  arc A14 (-43.577, 95.5303) -> (-48.7014, 93.0224) centre (0, 0) ccw
  arc A15 (-48.7014, 93.0224) -> (-92.5543, 49.5852) centre (0, 0) ccw construction
  arc A16 (92.5543, 49.5852) -> (48.7014, 93.0224) centre (0, 0) ccw construction
  arc A17 (92.5543, -49.5852) -> (92.5543, 49.5852) centre (0, 0) ccw construction
  arc A18 (48.7014, -93.0224) -> (92.5543, -49.5852) centre (0, 0) ccw construction
  arc A19 (-48.7014, -93.0224) -> (48.7014, -93.0224) centre (0, 0) ccw construction
  arc A20 (-92.5543, -49.5852) -> (-48.7014, -93.0224) centre (0, 0) ccw construction
  arc A21 (-92.5543, 49.5852) -> (-92.5543, -49.5852) centre (0, 0) ccw construction
  circle A22 centre (0, 0) radius 35 construction
  arc A23 (28.0199, 71.0163) -> (-28.0199, 71.0163) centre (0, 104.941) ccw construction
  line L44 (-83.085, 34.2947) -> (-90.6891, 41.8987)
  line L45 (-93.5297, 47.6709) -> (-92.5543, 49.5852) construction
  line L46 (-37.3889, 72.9198) -> (-76.014, 34.2947)
  arc A24 (-83.085, 34.2947) -> (-76.014, 34.2947) centre (-79.5495, 37.8302) ccw
  line L47 (-30.6393, 73.2144) -> (-28.0199, 71.0163)
  arc A25 (-30.6393, 73.2144) -> (-37.3889, 72.9198) centre (-33.8534, 69.3842) ccw
  arc A26 (-90.6891, 41.8987) -> (-87.3563, 48.4654) centre (0, 0) ccw construction
  arc A27 (44.1942, 83.085) -> (44.1942, 76.014) centre (47.7297, 79.5495) ccw
  line L48 (44.1942, 76.014) -> (76.014, 44.1942)
  arc A28 (76.014, 44.1942) -> (83.085, 44.1942) centre (79.5495, 47.7297) ccw
  line L49 (83.085, 34.2947) -> (90.6891, 41.8987)
  line L50 (37.3889, 72.9198) -> (76.014, 34.2947)
  arc A29 (76.014, 34.2947) -> (83.085, 34.2947) centre (79.5495, 37.8302) ccw
  arc A30 (37.3889, 72.9198) -> (30.6393, 73.2144) centre (33.8534, 69.3842) ccw
  arc A31 (5.5413, 61.2914) -> (28.0199, 71.0163) centre (0, 104.941) ccw
  arc A32 (-28.0199, 71.0163) -> (5.5413, 61.2914) centre (0, 104.941) ccw
  line L51 (30.6393, 73.2144) -> (28.0199, 71.0163)
  arc A33 (-87.3563, 48.4654) -> (-90.6891, 41.8987) centre (0, 0) ccw
  line L52 (83.085, 44.1942) -> (87.3563, 48.4654)
  arc A34 (90.6891, 41.8987) -> (87.3563, 48.4654) centre (0, 0) ccw
  line L53 (-44.1942, 83.085) -> (-48.6736, 87.5645)
  line L54 (44.0271, 95.3237) -> (43.577, 95.5303)
  line L55 (48.6736, 87.5645) -> (44.1942, 83.085)
  line L56 (0, 104.941) -> (-23.6028, 54.3247) construction
  point P0 (0, 95.941)
  point P1 (0, 105)
  point P2 (40.6586, 79.5495)
  point P3 (79.5495, 40.6586)
  point P4 (60.1041, 60.1041)
  point P5 (-87.5645, 48.6736)
  point P6 (-34.9935, 86.0061)
  point P7 (-23.542, 76.3968)
  point P8 (-94.5192, 45.7288)
  point P9 (-13.2817, 58.6489)
  point P10 (-28.5452, 71.4571)
  point P11 (13.2817, 58.6489)
  point P12 (-15.6369, 71.4076)
  dimension "d21" = 44.5856
  dimension "d0" = 74
  dimension "d1" = 100
  dimension "d2" = 28
  dimension "d3" = 15
  dimension "d4" = 45
  dimension "d5" = 55
  dimension "d6" = 16.3348
  dimension "d7" = 27.5
  dimension "d8" = 5
  dimension "d9" = 5
  dimension "d12" = 1
  dimension "d13" = 1.5
  dimension "d14" = 1.5
  dimension "d15" = 1
  dimension "d16" = 4
  dimension "d17" = 70
  dimension "d18" = 85
  dimension "d19" = 105
  dimension "d20" = 1.3619
  dimension "d22" = 88
  dimension "d23" = 7
  dimension "d25" = 5
  dimension "d26" = 7
  dimension "d27" = 5
  dimension "d83" = 7
  dimension "d84" = 5
  dimension "d85" = 5.1
  constraints: 87 point on circle, 76 end point, 34 centre point, 25 symmetric about line, 19 coincident, 18 point on line, 11 tangent, 6 collinear, 5 parallel, 4 midpoint, 4 vertical, 3 perpendicular, 1 concentric, 1 equal radius, 67 other
  measures "d0" diameter of A1
  measures "d1" angle of L2 L1
  measures "d2" distance from line of L4 A1.end
  measures "d3" distance of L1.end L40.end
  measures "d4" angle of L0 L5
  measures "d5" distance of point (40.659, 79.55) point (79.55, 40.659)
  measures "d6" distance of L8.start point (79.55, 40.659)
  measures "d7" distance of point (40.659, 79.55) point (60.104, 60.104)
  measures "d8" radius of A2
  measures "d9" distance of L8.end L9.end
  measures "d12" distance of L11.start L11.end
  measures "d13" distance of L11.start L13.start
  measures "d14" distance of L15.start L15.end
  measures "d15" distance of L15.start L43.end
  measures "d16" distance of L8.end L21.end
  measures "d17" diameter of A22
  measures "d18" distance of point (60.104, 60.104) L5.start
  measures "d19" radius of A17
  measures "d20" distance from line of L3 L4.start
  measures "d22" diameter of A23
  measures "d23" distance between parallel lines of L23 L44
  measures "d25" radius of A5
  measures "d26" distance between parallel lines of L46 L22
  measures "d27" radius of A24
  measures "d83" distance between parallel lines of L2 L47
  measures "d84" radius of A25
  measures "d85" radial gap between concentric circles of A21 A26
extrude "catcher" add sketch "Эскиз1" along normal blind 30
sketch "Эскиз4" plane through (37.3889, 0, 72.9198) normal (-0.7071068, 0, -0.7071068) x (-0.7071068, 0, 0.7071068)
  line L0 (-25.1241, 0) -> (-25.1241, 30) construction
  line L1 (-2.6241, 30) -> (-47.6241, 30) construction
  circle A0 centre (-25.1241, 11.2) radius 3.75
  circle A1 centre (-25.1241, 11.2) radius 10.25
  line L2 (-35.3741, 11.2) -> (-14.8741, 11.2) construction
  circle A2 centre (-17.6241, 11.2) radius 1.45
  circle A3 centre (-32.6241, 11.2) radius 1.45
  circle A4 centre (-25.1241, 18.7) radius 1.45
  line L3 (-25.1241, -24.6133) -> (-25.1241, 51.0797) projected
  circle A5 centre (-25.1241, 3.7) radius 1.45
  point P0 (-25.1241, 0.95)
  dimension "d90" = 7.5
  dimension "d91" = 11.2
  dimension "d92" = 20.5
  dimension "d234" = 2.9
  dimension "d235" = 15
  dimension "d250" = 2.9
  dimension "d251" = 15
  constraints: 6 centre point, 4 end point, 4 point on line, 3 point on circle, 2 midpoint, 2 symmetric about line, 1 coincident, 1 horizontal, 2 other
  measures "d90" diameter of A0
  measures "d91" distance of L0.start A0.centre
  measures "d92" diameter of A1
  measures "d234" diameter of A2
  measures "d235" distance of A2.centre A3.centre
  measures "d250" diameter of A4
  measures "d251" distance of A5.centre A4.centre
extrude "Выдавливание2" cut sketch "Эскиз4" against normal blind 7 contours A0 L3 | L3 A0
extrude "Выдавливание3" cut sketch "Эскиз4" against normal blind 4 contours A0 L3 A4 A1 A5 | A0 L3 A5 A1 A4 | L3 A4 | A4 L3 | A5 L3 | L3 A5 | A2 | A3
extrude "Выдавливание21" cut sketch "Эскиз4" against normal blind 10 contours L3 A4 | A4 L3 | A5 L3 | L3 A5
sketch "Эскиз5" plane through (-76.014, 0, 34.2947) normal (0.7071068, 0, -0.7071068) x (-0.7071068, 0, -0.7071068)
  line L0 (-29.5, 0) -> (-29.5, 40) construction
  line L1 (-7, 40) -> (-52, 40) construction
  circle A0 centre (-29.5, 11.2) radius 3.8
  circle A1 centre (-29.5, 11.2) radius 10.3
  point P0 (-29.5, 0.9)
  dimension "d99" = 20.6
  dimension "d97" = 7.6
  dimension "d98" = 11.2
  constraints: 4 end point, 2 coincident, 2 point on line, 1 centre point, 1 midpoint, 1 vertical, 1 vertical alignment, 2 other
  measures "d97" diameter of A0
  measures "d98" distance of L0.start A0.centre
ref_plane "РабПлоскость1" through (-23.7825, 0, 76.5969) normal (0, 0, -1) x (0, 1, 0)
sketch "Эскиз7" plane through (-23.7825, 0, 76.5969) normal (0, 0, -1) x (0, 1, 0)
  line L0 (0, 23.7825) -> (23, 23.7825) construction
  line L1 (28, 16.2825) -> (18, 16.2825)
  line L2 (18, 16.2825) -> (18, 31.2825)
  line L3 (18, 31.2825) -> (28, 31.2825)
  line L4 (28, 31.2825) -> (28, 16.2825)
  line L5 (28, 16.2825) -> (18, 31.2825) construction
  line L6 (18, 16.2825) -> (28, 31.2825) construction
  line L7 (31.15, 13.7825) -> (14.85, 13.7825) construction
  line L8 (14.85, 13.7825) -> (14.85, 33.7825) construction
  line L9 (14.85, 33.7825) -> (31.15, 33.7825) construction
  line L10 (31.15, 33.7825) -> (31.15, 13.7825) construction
  line L11 (31.15, 13.7825) -> (14.85, 33.7825) construction
  line L12 (14.85, 13.7825) -> (31.15, 33.7825) construction
  circle A0 centre (23, 23.7825) radius 10
  dimension "d107" = 23
  dimension "d108" = 10
  dimension "d109" = 15
  dimension "d238" = 16.3
  dimension "d239" = 20
  constraints: 26 end point, 4 midpoint, 4 parallel, 3 horizontal, 2 perpendicular, 1 centre point, 1 coincident, 1 tangent
  measures "d107" distance of L0.start L0.end
  measures "d108" distance of L2.end L3.end
  measures "d109" distance of L1.end L2.end
  measures "d238" distance of L8.end L9.end
  measures "d239" distance of L7.end L8.end
extrude "Выдавливание6" cut sketch "Эскиз7" along normal blind 20 contours L1 L2 L3 L4
sketch "Эскиз8" plane through (0, 0, 0) normal (0, 1, 0) x (-1, 0, 0)
  circle A0 centre (22.2621, 63.5478) radius 1.5 construction
  arc A1 (24.8591, 65.0496) -> (19.6651, 62.046) centre (22.2621, 63.5478) ccw construction
  line L0 (19.6651, 62.046) -> (18.23, 64.5276)
  line L1 (24.8591, 65.0496) -> (23.3668, 67.6303)
  arc A2 (19.6651, 62.046) -> (24.8591, 65.0496) centre (22.2621, 63.5478) ccw
  arc A3 (18.23, 64.5276) -> (23.3668, 67.6303) centre (-1.9905, 103.8071) ccw
  arc A4 (-23.7825, 76.5969) -> (23.7825, 76.5969) centre (0, 104.941) ccw construction
  line L2 (0, 67.941) -> (0, 60.941) construction
  line L3 (0, 60.941) -> (0, 79.7048) construction
  line L4 (22.2621, 63.5478) -> (20.8511, 65.9917) construction
  arc A5 (-28.0199, 71.0163) -> (28.0199, 71.0163) centre (0, 104.941) ccw construction
  arc A6 (-28.0199, 71.0163) -> (28.0199, 71.0163) centre (0, 104.941) ccw construction
  arc A7 (-28.0199, 71.0163) -> (28.0199, 71.0163) centre (0, 104.941) ccw construction
  point P0 (0, 0)
  dimension "d112" = 3
  dimension "d113" = 6
  dimension "d118" = 30
  dimension "d119" = 6
  dimension "d121" = 47
  constraints: 13 point on circle, 10 end point, 5 centre point, 3 point on line, 2 coincident, 1 parallel, 1 tangent, 1 vertical
  measures "d112" diameter of A0
  measures "d113" diameter of A1
  measures "d118" angle of L3 L4
  measures "d119" distance between parallel lines of L1 L0
  measures "d121" distance of A0.centre A3.centre
ref_plane "РабПлоскость2" through (0, 15, 0) normal (0, 1, 0) x (1, 0, 0)
sketch "Эскиз11" plane through (0, 15, 0) normal (0, 1, 0) x (1, 0, 0)
  arc A0 (28.0199, -71.0163) -> (-28.0199, -71.0163) centre (0, -104.941) ccw construction
  arc A1 (28.0199, -71.0163) -> (-28.0199, -71.0163) centre (0, -104.941) ccw construction
  point P0 (0, 0)
  constraints: 2 point on circle, 1 centre point
sketch "Эскиз12" plane through (0, 15, 0) normal (0, 1, 0) x (1, 0, 0)
  arc A0 (28.0199, -71.0163) -> (-28.0199, -71.0163) centre (0, -104.941) ccw construction
  arc A1 (23.7825, -76.5969) -> (-23.7825, -76.5969) centre (0, -104.941) ccw construction
  line L0 (0, -104.941) -> (-22.6617, -67.2257) construction
  line L1 (0, -104.941) -> (0, -60.941) construction
  line L2 (0, -104.941) -> (-26.5165, -60.8101) construction
  circle A2 centre (-24.2068, -64.6542) radius 1.55
  arc A3 (-26.7783, -66.1993) -> (-21.6353, -63.109) centre (-24.2068, -64.6542) ccw construction
  line L3 (-20.0374, -65.7683) -> (-21.6353, -63.109)
  line L4 (-25.1804, -68.8585) -> (-26.7783, -66.1993)
  arc A4 (-25.7519, -62.0827) -> (-26.7783, -66.1993) centre (-24.2068, -64.6542) ccw
  arc A5 (-21.6353, -63.109) -> (-25.7519, -62.0827) centre (-24.2068, -64.6542) ccw
  arc A6 (-20.0374, -65.7683) -> (-25.1804, -68.8585) centre (0, -104.941) ccw
  point P0 (0, 0)
  point P1 (0, -60.941)
  point P2 (-28.0199, -71.0163)
  dimension "d122" = 31
  dimension "d123" = 3.1
  dimension "d124" = 6
  constraints: 14 point on circle, 10 end point, 5 centre point, 5 tangent, 3 coincident, 2 parallel, 2 point on line, 1 collinear, 1 vertical, 2 other
  measures "d122" angle of L0 L1
  measures "d123" diameter of A2
  measures "d124" diameter of A3
ref_plane "РабПлоскость3" through (0, 24, 104.941) normal (0, 1, 0) x (1, 0, 0)
sketch "Эскиз18" plane through (0, 0, 0) normal (0, 1, 0) x (-1, 0, 0)
  arc A0 (-28.0199, 71.0163) -> (28.0199, 71.0163) centre (0, 104.941) ccw construction
  arc A1 (-23.7825, 76.5969) -> (23.7825, 76.5969) centre (0, 104.941) ccw construction
  line L0 (0, 104.941) -> (20.8949, 60.6155) construction
  circle A2 centre (20.0208, 62.4698) radius 1.55 construction
  arc A3 (21.5111, 58.7128) -> (22.4142, 59.3148) centre (20.8949, 60.6155) ccw construction
  line L1 (20.8949, 60.6155) -> (21.7477, 58.8064) construction
  circle A4 centre (20.0208, 62.4698) radius 3.05 construction
  line L2 (20.0208, 62.4698) -> (20.274, 65.5093) construction
  line L3 (20.0208, 62.4698) -> (17.5151, 64.2088) construction
  line L4 (20.0208, 62.4698) -> (17.262, 61.1693) construction
  line L5 (20.0208, 62.4698) -> (19.7677, 59.4303) construction
  line L6 (20.0208, 62.4698) -> (22.5265, 60.7308) construction
  line L7 (20.0208, 62.4698) -> (22.7797, 63.7703) construction
  line L8 (20.274, 65.5093) -> (22.7797, 63.7703) construction
  line L9 (22.7797, 63.7703) -> (22.5265, 60.7308) construction
  line L10 (22.5265, 60.7308) -> (19.7677, 59.4303) construction
  line L11 (19.7677, 59.4303) -> (17.262, 61.1693) construction
  line L12 (17.262, 61.1693) -> (17.5151, 64.2088) construction
  line L13 (17.5151, 64.2088) -> (20.274, 65.5093) construction
  circle A5 centre (20.0208, 62.4698) radius 4.7399 construction
  point P0 (0, 0)
  point P1 (20.6817, 61.0678)
  dimension "d145" = 3.1
  dimension "d147" = 6.1
  dimension "d146" = 2.5
  dimension "d150" = 360
  constraints: 28 end point, 2 coincident, 2 parallel, 2 point on line, 1 centre point, 1 collinear, 1 perpendicular, 1 point on circle, 25 other
  measures "d146" distance of L1.end point (20.682, 61.068)